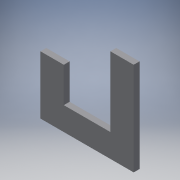
# Autodesk Inventor part: hook hook
Saved by Autodesk Inventor 2016 (Build 200138000, 138)
## iProperties
Created: 2016-03-29
Part Number: hook hook
Material: Generic
Document SubType Name: Modeling
Designer: gus
Density: 1 g/cm^3
Appearance: Default
Author: gus
Autodesk Inventor part; units mm, degrees
ref_plane "YZ Plane" through (0, 0, 0) normal (1, 0, 0) x (0, 1, 0)
ref_plane "XZ Plane" through (0, 0, 0) normal (0, 1, 0) x (-1, 0, 0)
ref_plane "XY Plane" through (0, 0, 0) normal (0, 0, 1) x (1, 0, 0)
sketch "Sketch1" plane through (0, 0, 0) normal (0, 0, 1) x (1, 0, 0)
  line L0 (0, 0) -> (0, -76.2)
  line L1 (0, -76.2) -> (-50.8, -76.2)
  line L2 (-50.8, -76.2) -> (-50.8, -38.1)
  line L3 (-50.8, -38.1) -> (-76.2, -38.1)
  line L4 (-76.2, -38.1) -> (-76.2, -101.6)
  line L5 (-76.2, -101.6) -> (25.4, -101.6)
  line L6 (25.4, -101.6) -> (25.4, 0)
  line L7 (0, 0) -> (25.4, 0)
  dimension "d0" = 101.6
  dimension "d1" = 25.4
  dimension "d2" = 25.4
  dimension "d3" = 25.4
  dimension "d4" = 50.8
  dimension "d5" = 76.2
  dimension "d6" = 63.5
  constraints: 16 end point, 4 perpendicular, 2 parallel, 1 vertical
  measures "d0" distance of L5.end L6.end
  measures "d1" distance of L2.end L3.end
  measures "d2" distance between parallel lines of L6 L0
  measures "d3" distance between parallel lines of L5 L1
  measures "d4" distance of L0.end L1.end
  measures "d5" distance of L0.start L0.end
  measures "d6" distance of L3.end L4.end
extrude "Extrusion1" add sketch "Sketch1" along normal blind 6.35
body "Solid1"
